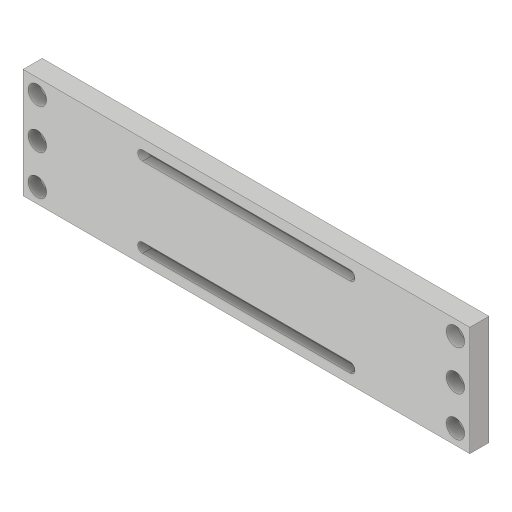
# Autodesk Inventor part: ASI_mesoSPIM_Bridge
Saved by Autodesk Inventor 2023 (Build 270158000, 158)
## iProperties
Created: 2020-05-15
Part Number: ASI_mesoSPIM_Bridge
Material: Generic
Document SubType Name: Modeling
Designer: voigt
Density: 1 g/cm^3
Appearance: Default
Author: voigt
Autodesk Inventor part; units mm, degrees
ref_plane "YZ Plane" through (0, 0, 0) normal (1, 0, 0) x (0, 1, 0)
ref_plane "XZ Plane" through (0, 0, 0) normal (0, 1, 0) x (-1, 0, 0)
ref_plane "XY Plane" through (0, 0, 0) normal (0, 0, 1) x (1, 0, 0)
sketch "Sketch1" plane through (0, 0, 0) normal (0, 0, 1) x (1, 0, 0)
  line L0 (-201.9864, -0.0159) -> (-218.1154, -0.0159) construction
  line L1 (-201.9864, -68.5959) -> (-218.1154, -68.5959) construction
  circle A0 centre (-234.0413, -9.3123) radius 2.5 construction
  circle A1 centre (-234.0413, -34.3059) radius 2.5 construction
  circle A2 centre (-234.0413, -59.2995) radius 2.5 construction
  line L2 (0.4039, -68.5877) -> (16.5329, -68.5877) construction
  line L3 (0.4039, -0.0077) -> (16.5329, -0.0077) construction
  circle A3 centre (27.9587, -59.2913) radius 2.5 construction
  circle A4 centre (27.9587, -34.2977) radius 2.5 construction
  circle A5 centre (27.9587, -9.3041) radius 2.5 construction
  line L4 (-243.0413, -0.0159) -> (36.9587, -0.0159)
  line L5 (36.9587, -0.0159) -> (36.9587, -68.5959)
  line L6 (36.9587, -68.5959) -> (-243.0413, -68.5959)
  line L7 (-243.0413, -68.5959) -> (-243.0413, -0.0159)
  line L8 (-103.0413, -534.726) -> (-103.0413, 430.7972) construction
  point P0 (0, 0)
  dimension "w" = 280
  dimension "d23" = 140
  dimension "d" = 262
  dimension "d34" = 131
  constraints: 18 end point, 6 centre point, 4 vertical alignment, 2 collinear, 2 parallel, 1 horizontal, 1 perpendicular, 1 vertical, 2 other
  measures "w" distance between parallel lines of L5 L7
  measures "d23" distance between parallel lines of L7 L8
  measures "d" distance of A5.centre A0.centre
  measures "d34" distance from line of L8 A0.centre
extrude "Extrusion1" add sketch "Sketch1" along normal blind 12
sketch "Sketch4" plane through (0, 0, 0) normal (0, 0, -1) x (-1, 0, 0)
  circle A0 centre (65.5413, -59.3059) radius 2.5 construction
  circle A1 centre (40.5413, -59.3059) radius 2.5 construction
  circle A2 centre (140.5413, -9.3059) radius 2.5 construction
  circle A3 centre (115.5413, -9.3059) radius 2.5 construction
  line L0 (40.5413, -59.3059) -> (172.5963, -59.3059) construction
  line L1 (167.5124, -9.3059) -> (3.0086, -9.3059) construction
  line L2 (243.0413, -0.0159) -> (-36.9587, -0.0159) construction
  line L3 (38.0413, -9.3059) -> (168.0413, -9.3059) construction
  line L4 (38.0413, -12.3559) -> (168.0413, -12.3559)
  line L5 (168.0413, -6.2559) -> (38.0413, -6.2559)
  arc A4 (38.0413, -6.2559) -> (38.0413, -12.3559) centre (38.0413, -9.3059) ccw
  arc A5 (168.0413, -12.3559) -> (168.0413, -6.2559) centre (168.0413, -9.3059) ccw
  line L6 (103.0413, 455.7975) -> (103.0413, -509.7257) construction
  line L7 (38.0413, -59.3059) -> (168.0413, -59.3059) construction
  line L8 (38.0413, -62.3559) -> (168.0413, -62.3559)
  line L9 (168.0413, -56.2559) -> (38.0413, -56.2559)
  arc A6 (38.0413, -56.2559) -> (38.0413, -62.3559) centre (38.0413, -59.3059) ccw
  arc A7 (168.0413, -62.3559) -> (168.0413, -56.2559) centre (168.0413, -59.3059) ccw
  point P0 (0, 0)
  point P1 (-36.9587, -0.0159)
  point P2 (103.0413, -9.3059)
  point P3 (103.0413, -59.3059)
  dimension "d10" = 9.29
  dimension "d11" = 6.1
  dimension "d12" = 65
  dimension "d13" = 65
  dimension "d14" = 6.1
  dimension "d15" = 65
  dimension "d16" = 65
  constraints: 22 end point, 8 point on circle, 8 tangent, 4 centre point, 3 point on line, 2 horizontal, 2 midpoint, 2 parallel, 1 horizontal alignment, 1 vertical, 4 other
  measures "d11" diameter of A5
  measures "d12" distance from line of L3.end L6
  measures "d13" distance from line of L6 L3.start
  measures "d14" diameter of A7
  measures "d15" distance from line of L6 L7.start
  measures "d16" distance from line of L6 L7.end
extrude "Extrusion2" cut sketch "Sketch4" against normal blind 12
sketch "Sketch5" plane through (0, 0, 0) normal (0, 0, -1) x (-1, 0, 0)
  line L0 (45.6373, -31.0674) -> (77.6413, -31.0674) construction
  arc A0 (168.0413, -12.3559) -> (168.0413, -6.2559) centre (168.0413, -9.3059) ccw construction
  arc A1 (168.0413, -62.3559) -> (168.0413, -56.2559) centre (168.0413, -59.3059) ccw construction
  arc A2 (38.0413, -6.2559) -> (38.0413, -12.3559) centre (38.0413, -9.3059) ccw construction
  arc A3 (38.0413, -56.2559) -> (38.0413, -62.3559) centre (38.0413, -59.3059) ccw construction
  line L1 (38.0413, -9.3059) -> (168.0413, -9.3059) construction
  line L2 (-36.9587, -0.0159) -> (243.0413, -0.0159) projected
  line L3 (38.0413, -14.5559) -> (168.0413, -14.5559)
  line L4 (168.0413, -4.0559) -> (38.0413, -4.0559)
  arc A4 (38.0413, -4.0559) -> (38.0413, -14.5559) centre (38.0413, -9.3059) ccw
  arc A5 (168.0413, -14.5559) -> (168.0413, -4.0559) centre (168.0413, -9.3059) ccw
  line L5 (38.0413, -59.3059) -> (168.0413, -59.3059) construction
  line L6 (38.0413, -64.5559) -> (168.0413, -64.5559)
  line L7 (168.0413, -54.0559) -> (38.0413, -54.0559)
  arc A6 (38.0413, -54.0559) -> (38.0413, -64.5559) centre (38.0413, -59.3059) ccw
  arc A7 (168.0413, -64.5559) -> (168.0413, -54.0559) centre (168.0413, -59.3059) ccw
  point P0 (0, 0)
  point P1 (243.0413, -0.0159)
  point P2 (103.0413, -9.3059)
  point P3 (103.0413, -59.3059)
  dimension "d19" = 10.5
  dimension "d20" = 10.5
  constraints: 16 end point, 8 point on circle, 8 tangent, 4 centre point, 3 parallel, 2 midpoint, 1 horizontal, 1 other
  measures "d19" diameter of A5
  measures "d20" diameter of A7
extrude "Extrusion3" cut sketch "Sketch5" against normal blind 6.5
sketch "Sketch6" plane through (0, 0, 12) normal (0, 0, 1) x (1, 0, 0)
  line L0 (-103.0413, -534.726) -> (-103.0413, 430.7972) construction
  point P0 (0, 0)
  point P1 (27.9587, -59.3064)
  point P2 (27.9587, -34.3064)
  point P3 (27.9587, -9.3064)
  point P4 (-234.0413, -59.3147)
  point P5 (-234.0413, -34.3147)
  point P6 (-234.0413, -9.3147)
  dimension "d36" = 25
  dimension "d37" = 262
  dimension "d38" = 131
  constraints: 4 vertical alignment
  measures "d36" distance of point (27.959, -34.306) point (27.959, -9.306)
  measures "d37" distance of point (-234.041, -9.315) point (27.959, -9.306)
  measures "d38" distance from line of L0 point (-234.041, -9.315)
hole "Hole2" at (27.9587, -59.3064, 12) at (27.9587, -34.3064, 12) at (27.9587, -9.3064, 12) at (-234.0413, -59.3147, 12) at (-234.0413, -34.3147, 12) at (-234.0413, -9.3147, 12) direction (0, 0, -1) diameter 6.1 end through all counterbore diameter 11.5 counterbore depth 7
equation "\"d23\" = 0.5 * w"
equation "\"d34\" = 0.5 * d"
equation "\"d37\" = d"
equation "\"d38\" = 0.5 * d"
body "Solid1"
